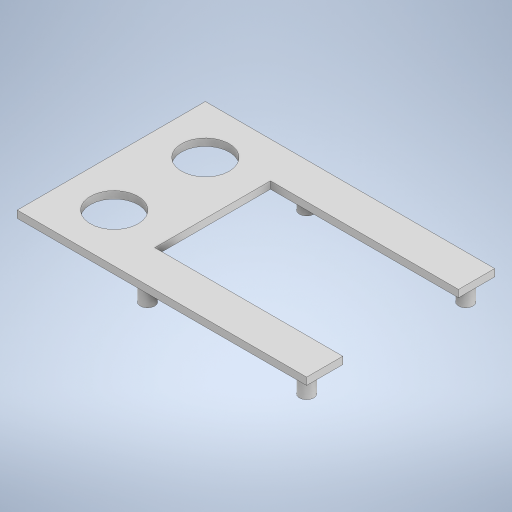
# Autodesk Inventor part: dust_cover
Saved by Autodesk Inventor 2023 (Build 270158000, 158)
## iProperties
Created: 2023-05-18
Part Number: dust_cover
Material: Generic
Document SubType Name: Modeling
Designer: mark
Density: 1 g/cm^3
Appearance: Default
Author: mark
Autodesk Inventor part; units mm, degrees
ref_plane "YZ Plane" through (0, 0, 0) normal (1, 0, 0) x (0, 1, 0)
ref_plane "XZ Plane" through (0, 0, 0) normal (0, 1, 0) x (-1, 0, 0)
ref_plane "XY Plane" through (0, 0, 0) normal (0, 0, 1) x (1, 0, 0)
sketch "Sketch1" plane through (0, 0, 0) normal (0, 1, 0) x (-1, 0, 0)
  line L0 (13.9277, -13.494) -> (-26.0723, -13.494)
  line L1 (-26.0723, -13.494) -> (-26.0723, 12.506)
  line L2 (-26.0723, 12.506) -> (13.9277, 12.506)
  line L3 (13.9277, 12.506) -> (13.9277, -13.494)
  point P0 (0, 0)
  dimension "d0" = 40
  dimension "d1" = 26
  constraints: 8 end point, 2 parallel, 1 horizontal, 1 perpendicular
  measures "d0" distance of L0.start L0.end
  measures "d1" distance of L2.end L0.start
extrude "Extrusion1" add sketch "Sketch1" along normal blind 1
sketch "Sketch2" plane through (0, 0, 0) normal (0, -1, 0) x (1, 0, 0)
  circle A0 centre (24.0723, -11.494) radius 1
  line L0 (26.0723, -13.494) -> (-13.9277, -13.494) projected
  line L1 (26.0723, 12.506) -> (26.0723, -13.494) projected
  point P0 (0, 0)
  dimension "d4" = 2
  dimension "d5" = 2
  dimension "d6" = 2
  constraints: 1 centre point
  measures "d4" diameter of A0
  measures "d5" distance from line of L0 A0.centre
  measures "d6" distance from line of L1 A0.centre
extrude "Extrusion2" add sketch "Sketch2" along normal blind 3
pattern_linear "Rectangular Pattern1" count 2 spacing 22 along (-1, 0, 0) count 2 spacing 22 along (0, 0, 1) of "Extrusion2"
sketch "Sketch3" plane through (0, 1, 0) normal (0, 1, 0) x (1, 0, 0)
  line L0 (26.0723, -12.506) -> (26.0723, 13.494) projected
  line L1 (26.0723, 8.494) -> (0.0723, 8.494)
  line L2 (0.0723, 8.494) -> (0.0723, -7.506)
  line L3 (0.0723, -7.506) -> (26.0723, -7.506)
  line L4 (26.0723, -7.506) -> (26.0723, 8.494)
  line L5 (26.0723, 13.494) -> (-13.9277, 13.494) projected
  line L6 (-13.9277, -12.506) -> (26.0723, -12.506) projected
  circle A0 centre (-7.2277, 6.794) radius 3.3
  circle A1 centre (-7.2277, -5.806) radius 3.3
  line L7 (-13.9277, 13.494) -> (-13.9277, -12.506) projected
  point P0 (0, 0)
  dimension "d15" = 26
  dimension "d16" = 5
  dimension "d17" = 5
  dimension "d18" = 6.6
  dimension "d19" = 6.6
  dimension "d24" = 6.7
  dimension "d25" = 6.7
  dimension "d26" = 6.7
  dimension "d27" = 6.7
  constraints: 8 end point, 2 centre point, 2 parallel, 1 horizontal, 1 perpendicular, 1 point on line
  measures "d15" distance of L3.end L2.end
  measures "d16" distance between parallel lines of L5 L1
  measures "d17" distance between parallel lines of L6 L3
  measures "d18" diameter of A0
  measures "d19" diameter of A1
  measures "d24" distance from line of L5 A0.centre
  measures "d25" distance from line of L6 A1.centre
  measures "d26" distance from line of L7 A1.centre
  measures "d27" distance from line of L7 A0.centre
extrude "Extrusion3" cut sketch "Sketch3" against normal through all contours L3 L2 L1 L0 | A0 | A1
equation "\"d19\" = d18"
equation "\"d25\" = d24"
equation "\"d26\" = d25"
equation "\"d27\" = d24"
body "Solid1"
